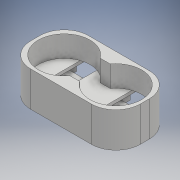
# Autodesk Inventor part: CaseBottom_CR123A
Saved by Autodesk Inventor 2018.1 (Build 221171000, 171)
## iProperties
Created: 2017-09-02
Part Number: CaseBottom_CR123A
Material: 一般
Document SubType Name: Modeling
Designer: sktom
Density: 1 g/cm^3
Appearance: 既定
Author: sktom
Autodesk Inventor part; units mm, degrees
ref_plane "YZ Plane" through (0, 0, 0) normal (1, 0, 0) x (0, 1, 0)
ref_plane "XZ Plane" through (0, 0, 0) normal (0, 1, 0) x (-1, 0, 0)
ref_plane "XY Plane" through (0, 0, 0) normal (0, 0, 1) x (1, 0, 0)
sketch "スケッチ4" plane through (0, 0, 0) normal (0, 0, 1) x (1, 0, 0)
  circle A0 centre (-8.5, 0) radius 8.5
  circle A1 centre (8.5, 0) radius 8.5
  line L0 (-17, -8.5) -> (17, -8.5)
  line L1 (17, -8.5) -> (17, 8.5)
  line L2 (17, 8.5) -> (-17, 8.5)
  line L3 (-17, 8.5) -> (-17, -8.5)
  line L4 (-18, 9.5) -> (18, 9.5)
  line L5 (18, 9.5) -> (18, -9.5)
  line L6 (18, -9.5) -> (-18, -9.5)
  line L7 (-18, -9.5) -> (-18, 9.5)
  line L8 (-1.6261, 5) -> (1.6261, 5)
  line L9 (-1.6261, -5) -> (1.6261, -5)
  point P0 (0, 0)
  dimension "d12" = 17
  dimension "d13" = 1
  dimension "d14" = 10
  constraints: 20 end point, 7 parallel, 5 point on circle, 5 tangent, 2 centre point, 2 horizontal alignment, 2 perpendicular, 1 equal radius, 1 horizontal, 3 other
  measures "d12" diameter of A1
  measures "d13" distance between parallel lines of L2 L4
  measures "d14" distance between parallel lines of L8 L9
extrude "押し出し4" add sketch "スケッチ4" along normal blind 10 contours A0 L2 A1 L8 | L9 A1 L0 A0 | A0 L3 L2 | L0 L3 A0 | L2 L1 A1 | A1 L1 L0 | L4 L5 L6 L7
sketch "スケッチ5" plane through (0, 0, 0) normal (0, 0, -1) x (-1, 0, 0)
  arc A0 (-1.6261, 5) -> (-1.6261, -5) centre (-8.5, 0) ccw projected
  line L0 (-1.6261, 5) -> (1.6261, 5) projected
  arc A1 (1.6261, -5) -> (1.6261, 5) centre (8.5, 0) ccw projected
  line L1 (1.6261, -5) -> (-1.6261, -5) projected
  line L2 (18, 9.5) -> (-18, 9.5) projected
  line L3 (-18, 9.5) -> (-18, -9.5) projected
  line L4 (-18, -9.5) -> (18, -9.5) projected
  line L5 (18, -9.5) -> (18, 9.5) projected
  point P0 (0, 0)
extrude "押し出し5" add sketch "スケッチ5" along normal blind 1.5 contours L0 A1 L1 A0 | L5 L4 L3 L2
sketch "スケッチ6" plane through (-18, 9.5, 10) normal (0, 1, 0) x (1, 0, 0)
  line L0 (16.3739, 10) -> (16.3739, 10) construction
  line L1 (16.3739, 10) -> (16.3739, 0) construction
  line L2 (16.3739, 0) -> (16.3739, 0) construction
  line L3 (16.3739, 10) -> (16.3739, 0) construction
  line L4 (19.6261, 10) -> (19.6261, 10) construction
  line L5 (19.6261, 10) -> (19.6261, 0) construction
  line L6 (19.6261, 0) -> (19.6261, 0) construction
  line L7 (19.6261, 10) -> (19.6261, 0) construction
  line L8 (19.6261, 10) -> (19.6261, 10) construction
  line L9 (19.6261, 10) -> (16.3739, 10) construction
  line L10 (16.3739, 10) -> (16.3739, 10) construction
  line L11 (16.3739, 10) -> (19.6261, 10) construction
  line L12 (16.3739, 10) -> (1, 10) construction
  line L13 (1, 10) -> (1, 8) construction
  line L14 (1, 8) -> (18, 8) construction
  line L15 (16.3739, 8) -> (16.3739, 10) construction
  line L16 (35, 10) -> (35, 0) construction
  line L17 (19.6261, 10) -> (35, 10) construction
  line L18 (35, 10) -> (35, 8) construction
  line L19 (35, 8) -> (18, 8) construction
  line L20 (19.6261, 7.5) -> (19.6261, 10) construction
  line L21 (4.75, 10) -> (14.25, 10)
  line L22 (14.25, 10) -> (14.25, 8)
  line L23 (14.25, 8) -> (4.75, 8)
  line L24 (4.75, 8) -> (4.75, 10)
  line L25 (19.6261, 10) -> (35, 10) projected
  line L26 (21.75, 10) -> (31.25, 10)
  line L27 (31.25, 10) -> (31.25, 8)
  line L28 (31.25, 8) -> (21.75, 8)
  line L29 (21.75, 8) -> (21.75, 10)
  line L30 (1, 10) -> (18, 10)
  line L31 (18, 10) -> (18, 7)
  line L32 (18, 7) -> (1, 7)
  line L33 (1, 7) -> (1, 10)
  line L34 (35, 10) -> (18, 10)
  line L35 (18, 10) -> (18, 7)
  line L36 (18, 7) -> (35, 7)
  line L37 (35, 7) -> (35, 10)
  line L38 (6.75, 8) -> (12.25, 8)
  line L39 (12.25, 8) -> (12.25, 7)
  line L40 (12.25, 7) -> (6.75, 7)
  line L41 (6.75, 7) -> (6.75, 8)
  line L42 (23.75, 8) -> (29.25, 8)
  line L43 (29.25, 8) -> (29.25, 7)
  line L44 (29.25, 7) -> (23.75, 7)
  line L45 (23.75, 7) -> (23.75, 8)
  point P0 (26.5, 8)
  point P1 (9.5, 8)
  dimension "d19" = 2
  dimension "d20" = 9.5
  dimension "d21" = 1
  dimension "d22" = 5.5
  constraints: 64 end point, 16 parallel, 14 point on line, 8 horizontal, 8 midpoint, 8 perpendicular, 4 collinear
  measures "d19" distance between parallel lines of L14 L12
  measures "d20" distance of L22.end L23.end
  measures "d21" distance between parallel lines of L19 L36
  measures "d22" distance of L38.start L38.end
extrude "押し出し6" cut sketch "スケッチ6" against normal blind 18 contours L21 L22 L23 L24 | L23 L39 L32 L41 | L45 L28 L43 L36 | L25 L27 L28 L29
extrude "押し出し7" add sketch "スケッチ6" against normal blind 18 contours L24 L23 L41 L32 L33 L30 | L30 L31 L32 L39 L23 L22 | L34 L25 L29 L28 L45 L36 L31 | L43 L28 L27 L25 L37 L36
sketch "スケッチ7" plane through (0, 0, -1.5) normal (0, 0, -1) x (-1, 0, 0)
  line L0 (13.25, 9.5) -> (13.25, -8.5) construction
  line L1 (13.25, -8.5) -> (3.75, -8.5) construction
  line L2 (3.75, 9.5) -> (3.75, -8.5) construction
  line L3 (13.25, 9.5) -> (3.75, 9.5) construction
  line L4 (-13.25, 9.5) -> (-13.25, -8.5) construction
  line L5 (-3.75, 9.5) -> (-13.25, 9.5) construction
  line L6 (-3.75, 9.5) -> (-3.75, -8.5) construction
  line L7 (-3.75, -8.5) -> (-13.25, -8.5) construction
  line L8 (-3.75, 9.5) -> (-3.75, -8.5) projected
  line L9 (-13.25, 9.5) -> (-3.75, 9.5)
  line L10 (-3.75, 9.5) -> (-3.75, 6.5)
  line L11 (-3.75, 6.5) -> (-13.25, 6.5)
  line L12 (-13.25, 6.5) -> (-13.25, 9.5)
  line L13 (3.75, 9.5) -> (13.25, 9.5)
  line L14 (13.25, 9.5) -> (13.25, 6.5)
  line L15 (13.25, 6.5) -> (3.75, 6.5)
  line L16 (3.75, 6.5) -> (3.75, 9.5)
  point P0 (0, 0)
  dimension "d27" = 3
  constraints: 16 end point, 4 parallel, 3 point on line, 2 horizontal, 2 perpendicular
  measures "d27" distance between parallel lines of L3 L15
extrude "押し出し8" cut sketch "スケッチ7" against normal up to next
fillet "フィレット1" radius 8 4 edges at (18, 9.5, 4.25) (18, -9.5, 4.25) (-18, 9.5, 4.25) (-18, -9.5, 4.25)
